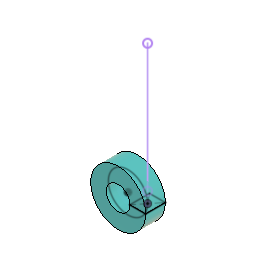
Lerdge.com Optical Endstop (Autodesk Fusion 360 archive; units mm, degrees)
design "Wiretie Cutout Donut"
Autodesk Fusion 360 part; units mm, degrees
sketch "Sketch1" plane through (0, 0, 0) normal (0, 0, 1) x (1, 0, 0)
  line L0 (-1.27, 1.5875) -> (1.27, 1.5875)
  line L1 (1.27, 1.5875) -> (1.27, -1.5875)
  line L2 (1.27, -1.5875) -> (-1.27, -1.5875)
  line L3 (-1.27, -1.5875) -> (-1.27, 1.5875)
  line L4 (-1.27, 1.5875) -> (1.27, -1.5875) construction
  line L5 (1.27, 1.5875) -> (-1.27, -1.5875) construction
  dimension "d4" = 2.54
  dimension "d5" = 3.175
  constraint horizontal L0
  constraint perpendicular L0 L1
  constraint parallel L0 L2
  constraint parallel L1 L3
  constraint coincident L4 origin
  constraint coincident L5 origin
  measures "d4" distance of L1.end L2.end
  measures "d5" distance of L0.end L1.end
sketch "Sketch2" plane through (0, 0, 0) normal (0, 1, 0) x (1, 0, 0)
  circle A0 centre (-3.175, 0) radius 3.175
  line L0 (0, -1.75) -> (0, -22.5)
  dimension "d6" = 6.35
  constraint tangent A0 L0
  constraint coincident A0 origin
  measures "d6" diameter of A0
sweep "Sweep1" add profiles "Sketch1" path "Sketch2" along A0 section 1
equation "WIDTH = 0.125 in" comment "Width of the torus box"
equation "DIAMETER = 0.25 in" comment "Diameter of the torus"
equation "d4 = HEIGHT"
equation "d5 = WIDTH"
equation "d6 = DIAMETER"
equation "HEIGHT = 0.1 in"

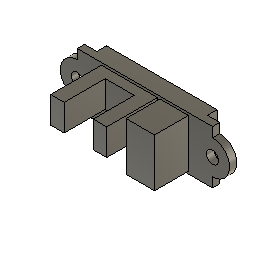
design "Lerdge.com Optical Endstop"
Autodesk Fusion 360 part; units mm, degrees
sketch "Sketch1" plane through (0, 0, 0) normal (0, 1, 0) x (1, 0, 0)
  line L0 (14, 5.5) -> (-14, 5.5)
  line L1 (-14, 5.5) -> (-14, 3.5)
  line L2 (-14, -3.5) -> (-14, -5.5)
  line L3 (-14, -5.5) -> (14, -5.5)
  line L4 (14, -5.5) -> (14, -3.5)
  line L5 (14, 5.5) -> (14, 3.5)
  arc A0 (14, -3.5) -> (14, 3.5) centre (14, 0) ccw
  arc A1 (-14, 3.5) -> (-14, -3.5) centre (-14, 0) ccw
  line L6 (-14, 0) -> (14, 0)
  line L7 (0, 0) -> (0, -21.2814)
  circle A2 centre (-14, 0) radius 1.25
  circle A3 centre (14, 0) radius 1.25
  line L8 (-9, -5) -> (-6.2, -5)
  line L9 (-6.2, -5) -> (-6.2, 0.5)
  line L10 (-6.2, 0.5) -> (-9, 0.5)
  line L11 (-9, 0.5) -> (-9, -5)
  line L12 (-0.2, -5) -> (2.6, -5)
  line L13 (2.6, -5) -> (2.6, 0.5)
  line L14 (2.6, 0.5) -> (-0.2, 0.5)
  line L15 (-0.2, 0.5) -> (-0.2, -5)
  line L16 (3.1, -5) -> (9, -5)
  line L17 (9, -5) -> (9, 5)
  line L18 (9, 5) -> (3.1, 5)
  line L19 (3.1, 5) -> (3.1, -5)
  line L20 (-17.5, 5.5) -> (17.5, 5.5) construction
  line L21 (17.5, 5.5) -> (17.5, -5.5) construction
  line L22 (17.5, -5.5) -> (-17.5, -5.5) construction
  line L23 (-17.5, -5.5) -> (-17.5, 5.5) construction
  line L24 (-6.2, 0.5) -> (-0.2, 0.5)
  line L25 (-6.2, -5) -> (-0.2, -5)
  line L26 (-11.4467, 5.5) -> (-11.4467, -5.5)
  line L27 (11.4467, 5.5) -> (11.4467, -5.5)
  line L28 (-14, -2.25) -> (14, -2.25) construction
  dimension "d2" = 11
  dimension "d3" = 28
  dimension "d4" = 3.5
  dimension "d5" = 2.5
  dimension "d6" = 0.5
  dimension "d9" = 0.5
  dimension "d12" = 0.5
  dimension "d13" = 0.5
  dimension "d14" = 5
  dimension "d19" = 17.7
  dimension "d20" = 2.8
  dimension "d21" = 11.3
  dimension "d22" = 35
  dimension "d27" = 2.5533
  constraint horizontal L0
  constraint perpendicular L0 L1
  constraint vertical L2
  constraint perpendicular L2 L3
  constraint perpendicular L3 L4
  constraint perpendicular L0 L5
  constraint equal L0 L3
  constraint equal L1 L2
  constraint equal L2 L4
  constraint equal L4 L5
  constraint collinear L1 L2
  constraint coincident L1.end A1.start
  constraint coincident L5.end A0.end
  constraint coincident A1.centre L6.start
  constraint coincident A0.centre L6.end
  constraint coincident L7.start L6
  constraint coincident L7.start origin
  constraint perpendicular L6 L7
  constraint midpoint L7.start L6
  constraint equal L3 L6
  constraint symmetric L2.end L3.end L7
  constraint concentric A1 A2
  constraint symmetric L7 A2 A3
  constraint horizontal L8
  constraint vertical L9
  constraint horizontal L10
  constraint vertical L11
  constraint horizontal L12
  constraint vertical L13
  constraint horizontal L14
  constraint vertical L15
  constraint collinear L10 L14
  constraint collinear L8 L12
  constraint equal L8 L12
  constraint horizontal L16
  constraint vertical L17
  constraint horizontal L18
  constraint vertical L19
  constraint collinear L12 L16
  constraint horizontal L20
  constraint vertical L21
  constraint horizontal L22
  constraint vertical L23
  constraint collinear L0 L20
  constraint collinear L3 L22
  constraint tangent A1 L23
  constraint tangent A0 L21
  constraint coincident L0 L26.start
  constraint coincident L20 L26.start
  constraint coincident L3 L26.end
  constraint coincident L22 L26.end
  constraint vertical L26
  constraint symmetric L7 L26.start L27.start
  constraint symmetric L7 L26.end L27.end
  constraint perpendicular L27 L28
  constraint coincident L2 L28.start
  constraint coincident L4 L28.end
  constraint symmetric L24 L25 L28
  measures "d2" distance of L0 L3
  measures "d3" distance of A0.centre A1.centre
  measures "d4" radius of A0
  measures "d5" diameter of A2
  measures "d6" distance of L3 L8
  measures "d9" distance of A1.centre L10
  measures "d12" distance of L0 L18
  measures "d13" distance of L13 L19
  measures "d14" distance of L4 L17
  measures "d19" distance of L15 L21
  measures "d20" distance of L8.start L8.end
  measures "d21" distance of L9 L23
  measures "d22" distance of L21 L23
  measures "d27" distance of A1.centre L26
extrude "Extrude1" add sketch "Sketch1" against normal blind 1.5 contours L0 L3 L4 L5 A0 L27 | L0 L6 L10 L11 L13 L14 L17 L18 L19 L24 L26 L27 | L0 L1 L2 L3 A1 L26 | L3 L6 L7 L12 L13 L16 L17 L19 L27 | L3 L6 L7 L8 L11 L12 L25 L26 | L6 L9 L15 L24 | L6 L9 L15 L25
extrude "Extrude2" add sketch "Sketch1" against normal blind 8.5 contours L6 L16 L17 L19 | L6 L17 L18 L19 | L6 L9 L10 L11 | L6 L8 L9 L11 | L6 L7 L12 L13 | L6 L13 L14 L15 | L6 L7 L12 L15
extrude "Extrude3" add sketch "Sketch1" against normal blind 12 contours L6 L9 L10 L11 | L6 L8 L9 L11 | L6 L7 L12 L13 | L6 L13 L14 L15 | L6 L7 L12 L15
extrude "Extrude4" add sketch "Sketch1" against normal blind 3.5 contours L6 L9 L15 L24 | L6 L9 L15 L25
extrude "Extrude5" add sketch "Sketch1" along normal blind 2 contours L0 L6 L10 L11 L13 L14 L17 L18 L19 L24 L26 L27 | L3 L6 L7 L12 L13 L16 L17 L19 L27 | L3 L6 L7 L8 L11 L12 L25 L26 | L6 L16 L17 L19 | L6 L17 L18 L19 | L6 L9 L10 L11 | L6 L8 L9 L11 | L6 L9 L15 L24 | L6 L9 L15 L25 | L6 L7 L12 L13 | L6 L13 L14 L15 | L6 L7 L12 L15
